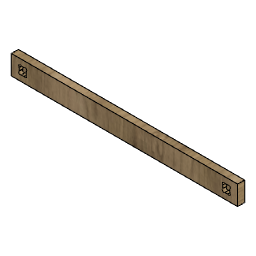
saeti_bak (Autodesk Fusion 360 design; units mm, degrees)
Autodesk Fusion 360 part; units mm, degrees
note: some values were not read from the file. Set by a fixed rule: which sketch regions a step uses.
sketch "Sketch6" plane through (0, 0, 0) normal (0, 1, 0) x (1, 0, 0)
  line L0 (0, 0) -> (580, 0)
  line L1 (580, 0) -> (580, -50)
  line L2 (580, -50) -> (0, -50)
  line L3 (0, -50) -> (0, 0)
  dimension "d24" = 580
  dimension "d25" = 50
  constraint horizontal L0
  constraint vertical L1
  constraint horizontal L2
  constraint vertical L3
  constraint coincident L0.start L3.end
  measures "d24" distance of L0.start L0.end
  measures "d25" distance of L0.start L2.end
extrude "Extrude4" add sketch "Sketch6" along normal blind 18
sketch "Sketch7" plane through (0, 0, 0) normal (0, -1, 0) x (1, 0, 0)
  line L0 (580, 0) -> (580, 50)
  line L1 (560, 35) -> (547.3517, 35)
  line L2 (542, 29.0536) -> (542, 20.9464)
  line L3 (547.3517, 15) -> (554.6483, 15)
  line L4 (560, 20.9464) -> (560, 29.0536)
  line L5 (32.6483, 35) -> (25.3517, 35)
  line L6 (38, 20.9464) -> (38, 29.0536)
  line L7 (25.3517, 15) -> (32.6483, 15)
  line L8 (20, 29.0536) -> (20, 20.9464)
  arc A0 (25.3517, 35) -> (20, 29.0536) centre (22.6759, 32.0268) ccw
  arc A1 (38, 29.0536) -> (32.6483, 35) centre (35.3241, 32.0268) ccw
  arc A2 (32.6483, 15) -> (38, 20.9464) centre (35.3241, 17.9732) ccw
  arc A3 (20, 20.9464) -> (25.3517, 15) centre (22.6759, 17.9732) ccw
  arc A4 (560, 29.0536) -> (554.6483, 35) centre (557.3241, 32.0268) ccw
  arc A5 (547.3517, 35) -> (542, 29.0536) centre (544.6759, 32.0268) ccw
  arc A6 (542, 20.9464) -> (547.3517, 15) centre (544.6759, 17.9732) ccw
  arc A7 (554.6483, 15) -> (560, 20.9464) centre (557.3241, 17.9732) ccw
  dimension "d48" = 8
  dimension "d49" = 8
  dimension "d50" = 8
  dimension "d51" = 8
  dimension "d54" = 8
  dimension "d55" = 8
  dimension "d56" = 8
  dimension "d57" = 8
  constraint horizontal L1
  constraint vertical L2
  constraint horizontal L3
  constraint vertical L4
  constraint coincident L1.start A4
  constraint horizontal L5
  constraint vertical L8
  constraint horizontal L7
  constraint vertical L6
  constraint coincident L1 A4.end
  measures "d48" diameter of A5
  measures "d49" diameter of A4
  measures "d50" diameter of A6
  measures "d51" diameter of A7
  measures "d54" diameter of A0
  measures "d55" diameter of A1
  measures "d56" diameter of A3
  measures "d57" diameter of A2
extrude "Extrude7" cut sketch "Sketch7" against normal blind 10
equation "breidd_bak = 50 mm"
equation "t_bak = 18 mm"
equation "lengd_bak = 580 mm"
equation "d24 = lengd_bak"
equation "d25 = breidd_bak"
equation "d26 = t_bak"
equation "dog_r = 8 mm"
equation "d48 = dog_r"
equation "d49 = dog_r"
equation "d50 = dog_r"
equation "d51 = dog_r"
equation "d54 = dog_r"
equation "d55 = dog_r"
equation "d56 = dog_r"
equation "d57 = dog_r"
